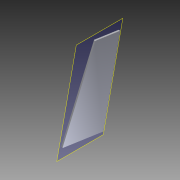
# Autodesk Inventor part: Panel_side
Saved by Autodesk Inventor 2013 (Build 170138000, 138)
## iProperties
Created: 2013-02-02
Part Number: Panel_side
Material: Aluminum 6061
Document SubType Name: Modeling
Designer: xylzlyx
Density: 1 g/cm^3
Author: xylzlyx
Autodesk Inventor part; units mm, degrees
ref_plane "YZ Plane" through (0, 0, 0) normal (1, 0, 0) x (0, 1, 0)
ref_plane "XZ Plane" through (0, 0, 0) normal (0, 1, 0) x (-1, 0, 0)
ref_plane "XY Plane" through (0, 0, 0) normal (0, 0, 1) x (1, 0, 0)
ref_plane "Work Plane1" through (-221.4413, -90.9255, -118.1004) normal (-0.9848078, 0.1736482, 0) x (-0.1736482, -0.9848078, 0)
sketch "Sketch1" plane through (-221.4413, -90.9255, -118.1004) normal (-0.9848078, 0.1736482, 0) x (-0.1736482, -0.9848078, 0)
  line L0 (0, 0) -> (-0.5513, 3.1268) construction
  line L1 (-0.5513, 3.1268) -> (245.7896, 46.5633) construction
  line L2 (245.7896, 46.5633) -> (246.341, 43.4366) construction
  line L3 (246.341, 43.4366) -> (0, 0) construction
  line L4 (254.4978, -57.6752) -> (251.371, -58.2265) construction
  line L5 (251.371, -58.2265) -> (233.8339, 41.2312) construction
  line L6 (233.8339, 41.2312) -> (236.9607, 41.7826) construction
  line L7 (236.9607, 41.7826) -> (254.4978, -57.6752) construction
  line L8 (12.5071, 2.2053) -> (23.1628, -58.2265) construction
  line L9 (23.1628, -58.2265) -> (20.0361, -58.7779) construction
  line L10 (20.0361, -58.7779) -> (9.3803, 1.654) construction
  line L11 (9.3803, 1.654) -> (12.5071, 2.2053) construction
  line L12 (264.2669, -61.4015) -> (10.2669, -61.4015) construction
  line L13 (10.2669, -61.4015) -> (10.2669, -58.2265) construction
  line L14 (10.2669, -58.2265) -> (264.2669, -58.2265) construction
  line L15 (264.2669, -58.2265) -> (264.2669, -61.4015) construction
  line L16 (233.8339, 41.2312) -> (251.371, -58.2265)
  line L17 (251.371, -58.2265) -> (23.1628, -58.2265)
  line L18 (23.1628, -58.2265) -> (12.5071, 2.2053)
  line L19 (12.5071, 2.2053) -> (233.8339, 41.2312)
  point P0 (-127.997, 118.1004)
  constraints: 40 end point, 4 collinear, 2 horizontal, 2 vertical, 28 other
extrude "SidePanel" add sketch "Sketch1" against normal blind 3.175
fillet "Fillet1" radius 1 4 edges at (-263.5281, -338.7532, -176.327) (-260.4828, -321.4826, -76.8692) (-223.9001, -114.0121, -176.327) (-222.0498, -103.5182, -115.8951)
body "Solid1"
